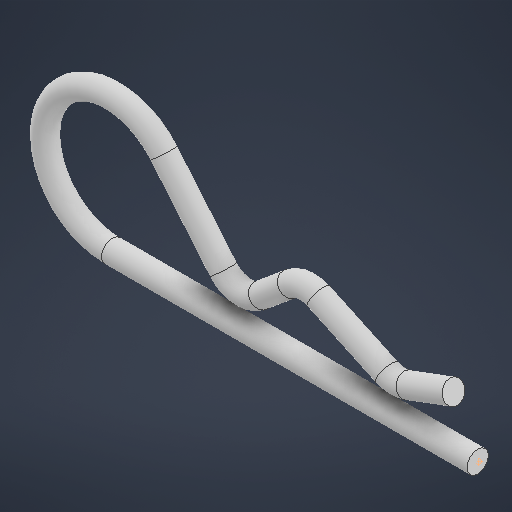
# Autodesk Inventor part: B1
Saved by Autodesk Inventor 2025.4 (Build 294407000, 407)
## iProperties
Created: 2026-05-10
Part Number: B1
Material: Generic
Document SubType Name: Modeling
Designer: VuQuan
Density: 1 g/cm^3
Appearance: Default
Author: VuQuan
Autodesk Inventor part; units mm, degrees
ref_plane "YZ Plane" through (0, 0, 0) normal (1, 0, 0) x (0, 1, 0)
ref_plane "XZ Plane" through (0, 0, 0) normal (0, 1, 0) x (-1, 0, 0)
ref_plane "XY Plane" through (0, 0, 0) normal (0, 0, 1) x (1, 0, 0)
sketch "Sketch1" plane through (0, 0, 0) normal (0, 0, 1) x (1, 0, 0)
  line L0 (0, 0) -> (-68, 0)
  arc A0 (-58.4163, 20.5251) -> (-68, 0) centre (-68, 12.5) ccw
  line L1 (-58.4163, 20.5251) -> (-47.3335, 7.2899)
  arc A1 (-47.3335, 7.2899) -> (-40.2899, 6.6665) centre (-43.5, 10.5) ccw
  line L2 (-40.2899, 6.6665) -> (-34.9101, 11.1715)
  arc A2 (-29.5895, 11.8708) -> (-34.9101, 11.1715) centre (-31.7, 7.338) ccw
  line L3 (-29.5895, 11.8708) -> (-16.9105, 5.9673)
  arc A3 (-16.9105, 5.9673) -> (-13.0552, 5.8143) centre (-14.8, 10.5) ccw
  line L4 (-13.0552, 5.8143) -> (-4.5, 9)
  dimension "d0" = 68
  dimension "d1" = 12.5
  dimension "d2" = 24.5
  dimension "d3" = 36.3
  dimension "d4" = 53.2
  dimension "d5" = 5
  dimension "d6" = 10.5
  dimension "d8" = 9
  dimension "d9" = 63.5
  constraints: 10 end point, 8 point on circle, 8 tangent, 4 centre point, 2 equal radius, 1 horizontal, 1 horizontal alignment, 1 perpendicular
  measures "d0" horizontal distance of L0.start A0.centre
  measures "d1" radius of A0
  measures "d2" horizontal distance of A1.centre A0.centre
  measures "d3" horizontal distance of A0.centre A2.centre
  measures "d4" horizontal distance of A0.centre A3.centre
  measures "d5" radius of A1
  measures "d6" distance from line of L0 A3.centre
  measures "d8" distance from line of L0 L4.end
  measures "d9" horizontal distance of A0.centre L4.end
sketch "Sketch2" plane through (0, 0, 0) normal (1, 0, 0) x (0, 1, 0)
  circle A0 centre (0, 0) radius 2
  dimension "d7" = 4
  constraints: 1 centre point, 1 coincident
  measures "d7" diameter of A0
sweep "Sweep1" add profiles "Sketch2" path "Sketch1"
body "Solid1"
